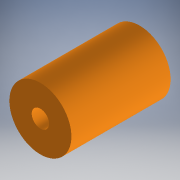
# Autodesk Inventor part: Motor Rotary Encoder Coupler
Saved by Autodesk Inventor 2018 (Build 220112000, 112)
## iProperties
Created: 2018-01-13
Part Number: Motor Rotary Encoder Coupler
Material: Generic
Document SubType Name: Modeling
Designer: Moochster
Density: 1 g/cm^3
Appearance: Orange
Author: Moochster
Autodesk Inventor part; units mm, degrees
ref_plane "YZ Plane" through (0, 0, 0) normal (1, 0, 0) x (0, 1, 0)
ref_plane "XZ Plane" through (0, 0, 0) normal (0, 1, 0) x (-1, 0, 0)
ref_plane "XY Plane" through (0, 0, 0) normal (0, 0, 1) x (1, 0, 0)
sketch "Sketch1" plane through (0, 0, 0) normal (0, 1, 0) x (-1, 0, 0)
  circle A0 centre (0, 0) radius 1.4
  circle A1 centre (0, 0) radius 5
  circle A2 centre (0, 0) radius 1.115
  dimension "d0" = 2.8
  dimension "d1" = 10
  constraints: 3 centre point, 2 coincident, 2 other
  measures "d0" diameter of A0
  measures "d1" diameter of A1
extrude "Extrusion1" add sketch "Sketch1" along normal blind 16 contours A0 | A1 | A2
extrude "Extrusion2" cut sketch "Sketch1" along normal blind 8 contours A0 | A2
sketch "Sketch2" plane through (0, 16, 0) normal (0, 1, 0) x (1, 0, 0)
  circle A0 centre (0, 0) radius 3 construction
  circle A1 centre (0, 0) radius 3.19
  line L0 (-2.8414, 1.45) -> (2.8414, 1.45) construction
  line L1 (-2.7421, 1.63) -> (2.7421, 1.63)
  point P0 (0, -3)
  dimension "d6" = 6
  dimension "d7" = 6.38
  dimension "d8" = 4.45
  dimension "d9" = 0.18
  constraints: 4 end point, 4 point on circle, 2 coincident, 2 horizontal, 2 vertical alignment, 1 centre point, 2 other
  measures "d7" diameter of A1
  measures "d8" distance from line of L0 point (0, -3)
  measures "d9" distance between parallel lines of L0 L1
extrude "Extrusion3" cut sketch "Sketch2" against normal blind 6 contours A1 L1 picked at (0.1058, 0.0286)
body "Solid1"
